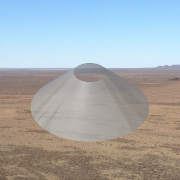
# Autodesk Inventor part: 2r5scs
Saved by Autodesk Inventor 2013 SP2 (Build 170200200, 200)
## iProperties
Company: HERA Project
Created: 2013-05-31
Part Number: 2r5scs
Material: Glass
Document SubType Name: Modeling
Designer: David DeBoer
Density: 2.18 g/cm^3
Description: Splash cone surface
Mass: 6287 g
Surface Area: 17122.3 cm^2
Volume: 2883.94 cm^3
Author: David DeBoer
Title: Splash
Autodesk Inventor part; units mm, degrees
ref_plane "YZ Plane" through (0, 0, 0) normal (1, 0, 0) x (0, 1, 0)
ref_plane "XY Plane" through (0, 0, 0) normal (0, 0, 1) x (1, 0, 0)
sketch "Sketch1" plane through (0, 0, 0) normal (0, 0, 1) x (1, 0, 0)
  line L0 (-457.2, 0) -> (0, 457.2)
  line L1 (-457.2, 0) -> (-46.77397, 0) construction
  line L2 (0, 452.386467) -> (-448.982785, 3.403682)
  line L3 (-448.982785, 3.403682) -> (-452.386467, 0)
  line L4 (-457.2, 0) -> (-452.386467, 0)
  line L5 (0, 457.2) -> (0, 452.386467)
  line L6 (0, 452.386467) -> (0, 0) construction
  point P0 (0, 0)
  dimension "d0" = 0
  dimension "d1" = 45
  constraints: 14 end point, 3 collinear, 1 horizontal, 1 perpendicular, 1 point on line
  measures "d0" horizontal distance of point (0, 0) L0.end
  measures "d1" angle of L1 L0
sketch "Sketch1 outline for Revolution1" plane through (0, 0, 0) normal (0, 0, 1) x (1, 0, 0)
  line L0 (0, 452.386467) -> (0, 457.2)
  line L1 (-448.982785, 3.403682) -> (0, 452.386467)
  line L2 (-452.386467, 0) -> (-448.982785, 3.403682)
  line L3 (-457.2, 0) -> (-452.386467, 0)
  line L4 (0, 457.2) -> (-457.2, 0)
revolve "Revolution1" add sketch "Sketch1 outline for Revolution1" angle 360 about axis through (0, 457.2, 0) along (0, -1, 0)
ref_plane "Work Plane1" through (0, 508, 0) normal (0, 1, 0) x (-1, 0, 0)
sketch "Sketch5" plane through (0, 508, 0) normal (0, 1, 0) x (-1, 0, 0)
  circle A0 centre (0, 0) radius 127
  dimension "d7" = 254
  constraints: 1 centre point, 1 coincident
  measures "d7" diameter of A0
sketch "Sketch5 outline for Extrusion2" plane through (0, 508, 0) normal (0, 1, 0) x (-1, 0, 0)
  circle A0 centre (0, 0) radius 127
extrude "Extrusion2" cut sketch "Sketch5 outline for Extrusion2" against normal blind 508
body "Solid1"
